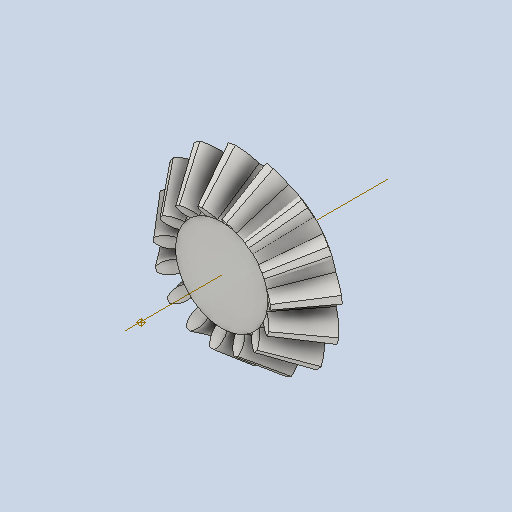
# Autodesk Inventor part: Bevel Gear2
Saved by Autodesk Inventor 2023 (Build 270158000, 158)
## iProperties
Created: 2023-02-02
Part Number: Bevel Gear2
Material: Steel, Mild
Document SubType Name: Modeling
Designer: MOHIKA
Categories: <?xml version="1.0" encoding="UTF-16"?> <MemberInstance><Categories><FamilyTemplate><FamilyTemplateParameter ValueType="xs:double" Id="1" ObjectReferenceKey="da_z" ObjectType="kUserParameterObject"/><FamilyTemplateParameter ValueType="xs:double" Id="2" ObjectReferenceKey="da_b" ObjectType="kUserParameterObject"/><FamilyTemplateParameter ValueType="xs:double" Id="3" ObjectReferenceKey="da_beta" ObjectType="kUserParameterObject"/><FamilyTemplateParameter ValueType="xs:double" Id="4" ObjectReferenceKey="da_dae" ObjectType="kUserParameterObject"/><FamilyTemplateParameter ValueType="xs:double" Id="5" ObjectReferenceKey="da_ve" ObjectType="kUserParameterObject"/><FamilyTemplateParameter ValueType="xs:double" Id="6" ObjectReferenceKey="da_omega" ObjectType="kUserParameterObject"/><FamilyTemplateParameter ValueType="xs:string" Id="7" ObjectReferenceKey="EAIAABAAAAAAHwAAAAAAAIAAAAAAAAAA" ObjectType="83914240" SubObjectId="SurfaceGeometry"/></FamilyTemplate><ParamToTemplateMap><ParamToTemplate CategoryParameter="//CategoryParameter[@InternalName='046C89C9-8512-4d59-83FE-43B91F4F132A']" TemplateParameter="1"/><ParamToTemplate CategoryParameter="//CategoryParameter[@InternalName='2552DF32-E462-4b46-AEBF-C6C7768E72AC']" TemplateParameter="2"/><ParamToTemplate CategoryParameter="//CategoryParameter[@InternalName='C9EE641D-15FC-4fae-A226-E94C4372FDD7']" TemplateParameter="3"/><ParamToTemplate><ParamToTemplate CategoryParameter="//CategoryParameter[@InternalName='00B6519A-459B-49c7-AD84-2E56D39A5744']" ConstantValue="-0.279412"/></ParamToTemplate><ParamToTemplate><ParamToTemplate CategoryParameter="//CategoryParameter[@InternalName='04B31F0E-C7A6-4894-AA32-9629BEFACF47']" ConstantValue="1.000000"/></ParamToTemplate><ParamToTemplate><ParamToTemplate CategoryParameter="//CategoryParameter[@InternalName='43CBEC2E-7847-49e7-A936-2F7889FCB2D9']" ConstantValue="0.200000"/></ParamToTemplate><ParamToTemplate><ParamToTemplate CategoryParameter="//CategoryParameter[@InternalName='B1EFC894-105D-4ebd-86BF-FA20ED196853']" ConstantValue="0.300000"/></ParamToTemplate><ParamToTemplate><ParamToTemplate CategoryParameter="//CategoryParameter[@InternalName='51175063-3D10-4879-93E8-6246FE8B403D']" ConstantValue="2060000000.000000"/></ParamToTemplate><ParamToTemplate><ParamToTemplate CategoryParameter="//CategoryParameter[@InternalName='A3A52E27-4454-46a9-B0BD-C932399B70AF']" ConstantValue="0.300000"/></ParamToTemplate><ParamToTemplate CategoryParameter="//CategoryParameter[@InternalName='2A200944-5A8C-41ca-B96E-8520D2E510F1']" TemplateParameter="4"/><ParamToTemplate><ParamToTemplate CategoryParameter="//CategoryParameter[@InternalName='1A637F62-92C8-44bc-B81F-10802510B579']" ConstantValue="1.557144"/></ParamToTemplate><ParamToTemplate CategoryParameter="//CategoryParameter[@InternalName='B52DD4BE-6863-48fb-BF58-89EF6F9EC65C']" TemplateParameter="5"/><ParamToTemplate><ParamToTemplate CategoryParameter="//CategoryParameter[@InternalName='3956BFF2-84D2-457d-93C2-9B0613DEBA67']" ConstantValue="0.922321"/></ParamToTemplate><ParamToTemplate CategoryParameter="//CategoryParameter[@InternalName='739CFA02-461B-4bf8-8049-181FCAD8B28F']" TemplateParameter="6"/><ParamToTemplate><ParamToTemplate CategoryParameter="//CategoryParameter[@InternalName='A27E999F-E2CE-4481-8A2A-EBF499C4C3C5']" ConstantValue="0.050000"/></ParamToTemplate><ParamToTemplate><ParamToTemplate CategoryParameter="//CategoryParameter[@InternalName='9E1B4470-B2D3-4ff1-B813-535BB4CDF51A']" ConstantValue="3520000.000000"/></ParamToTemplate><ParamToTemplate><ParamToTemplate CategoryParameter="//CategoryParameter[@InternalName='F8452263-BFF6-458c-9FB1-07C4B99E95CD']" ConstantValue="11400000.000000"/></ParamToTemplate><ParamToTemplate><ParamToTemplate CategoryParameter="//CategoryParameter[@InternalName='3E3BB259-FD49-497f-8171-6EBC954A3479']" ConstantValue="2.000000"/></ParamToTemplate><ParamToTemplate CategoryParameter="//CategoryParameter[@InternalName='27C3BAF2-7550-4e4b-AE2C-0DB134B7D9B7']" TemplateParameter="7"/></ParamToTemplateMap><Category DisplayName="Gear" InternalName="DC85795E-93AB-48d5-8EEE-5A27447B64BD" Mnemonic="Gear"><CategoryParameter DisplayName="z" InternalName="046C89C9-8512-4d59-83FE-43B91F4F132A" Mnemonic="z"/><CategoryParameter DisplayName="b" InternalName="2552DF32-E462-4b46-AEBF-C6C7768E72AC" Mnemonic="b"/><CategoryParameter DisplayName="||b|" InternalName="C9EE641D-15FC-4fae-A226-E94C4372FDD7" Mnemonic="beta"/><CategoryParameter DisplayName="x" InternalName="00B6519A-459B-49c7-AD84-2E56D39A5744" Mnemonic="x"/><CategoryParameter DisplayName="a*" InternalName="04B31F0E-C7A6-4894-AA32-9629BEFACF47" Mnemonic="a"/><CategoryParameter DisplayName="c*" InternalName="43CBEC2E-7847-49e7-A936-2F7889FCB2D9" Mnemonic="c"/><CategoryParameter DisplayName="r|.f|*" InternalName="B1EFC894-105D-4ebd-86BF-FA20ED196853" Mnemonic="rf"/><CategoryParameter DisplayName="E" InternalName="51175063-3D10-4879-93E8-6246FE8B403D" Mnemonic="E"/><CategoryParameter DisplayName="||m|" InternalName="A3A52E27-4454-46a9-B0BD-C932399B70AF" Mnemonic="mi"/><Category DisplayName="BevelGear" InternalName="0C98F69A-0C2B-4791-B2FE-7691BB227E77" Mnemonic="BevelGear"><CategoryParameter DisplayName="d|.ae|" InternalName="2A200944-5A8C-41ca-B96E-8520D2E510F1" Mnemonic="dae"/><CategoryParameter DisplayName="d|.ai|" InternalName="1A637F62-92C8-44bc-B81F-10802510B579" Mnemonic="dai"/><CategoryParameter DisplayName="A|.e|" InternalName="B52DD4BE-6863-48fb-BF58-89EF6F9EC65C" Mnemonic="ve"/><CategoryParameter DisplayName="A|.i|" InternalName="3956BFF2-84D2-457d-93C2-9B0613DEBA67" Mnemonic="vi"/><CategoryParameter DisplayName="||S|" InternalName="739CFA02-461B-4bf8-8049-181FCAD8B28F" Mnemonic="omega"/><CategoryParameter DisplayName="x|.t|" InternalName="A27E999F-E2CE-4481-8A2A-EBF499C4C3C5" Mnemonic="xt"/><CategoryParameter DisplayName="||s||.Flim|" InternalName="9E1B4470-B2D3-4ff1-B813-535BB4CDF51A" Mnemonic="sFlim"/><CategoryParameter DisplayName="||s||.Hlim|" InternalName="F8452263-BFF6-458c-9FB1-07C4B99E95CD" Mnemonic="sHlim"/><CategoryParameter DisplayName="type" InternalName="3E3BB259-FD49-497f-8171-6EBC954A3479" Mnemonic="type"/><CategoryParameter DisplayName="PitchDiameter" InternalName="27C3BAF2-7550-4e4b-AE2C-0DB134B7D9B7" Mnemonic="IDS_PITCHDIAM"/></Category></Category></Categories></MemberInstance>
Mass: 60.9118 g
Surface Area: 34.3074 cm^2
Volume: 7.7496 cm^3
Density: 7.86 g/cm^3
Appearance: Steel
CustomPartVersion: 1
Author: MOHIKA
Autodesk Inventor part; units mm, degrees
ref_plane "Mesh Plane2" through (0, 0, 0) normal (0.9781476, 0.2079117, 0) x (0, 0, 1)
sketch "Teeth Body Sketch" plane through (0, 0, 0) normal (1, 0, 0) x (0, 1, 0)
  line L0 (0, 0) -> (9.474706, -16.331471) construction
  line L1 (9.474706, -16.331471) -> (12.114706, -14.351471)
  line L2 (12.114706, -14.351471) -> (0, 0) construction
  line L3 (11.25, -15) -> (0, 0) construction
  line L4 (6.089078, -10.495692) -> (7.785718, -9.223212)
  line L5 (9.474706, -16.331471) -> (6.089078, -10.495692)
  line L6 (12.114706, -14.351471) -> (7.785718, -9.223212)
  line L7 (0, -39.386751) -> (0, 6.564458)
  line L8 (0, -15) -> (12.114706, -15) construction
  dimension "d0" = 22.5
  dimension "d1" = 18.94941
  dimension "d2" = 24.22941
  dimension "d3" = 6.7
  dimension "d4" = 14.35147
  constraints: 16 end point, 4 point on line, 3 perpendicular, 2 collinear, 1 horizontal alignment, 1 vertical alignment
  measures "d0" diameter of L3.start L7
  measures "d1" diameter of L0.end L7
  measures "d2" diameter of L1.end L7
  measures "d3" distance between parallel lines of L1 L4
  measures "d4" vertical distance of L1.end L0.start
revolve "Teeth Body" add sketch "Teeth Body Sketch" angle 360 about axis through (0, 0, 0) along (0, 0, 1)
ref_plane "Tooth Plane" through (0, 11.25, -15) normal (0, -0.6, 0.8) x (1, 0, 0)
sketch "Start Sketch" plane through (0, 11.25, -15) normal (0, -0.6, 0.8) x (1, 0, 0)
  line L0 (0, -23.505131) -> (0, 10.644758)
  arc A0 (-0.947228, -2.615118) -> (-3.205708, 1.749187) centre (-4.944424, -1.917101) ccw
  arc A1 (3.205708, 1.749187) -> (0.947228, -2.615118) centre (4.944424, -1.917101) ccw
  line L1 (-0.947228, -2.615118) -> (0.947228, -2.615118)
  arc A2 (3.205708, 1.749187) -> (-3.205708, 1.749187) centre (0, -14.0625) ccw
  dimension "d7" = 4.05768
  dimension "d8" = 4.94442
  dimension "d9" = 12.1454
  dimension "d57" = 16.13338
  dimension "d58" = 11.44738
  constraints: 6 point on circle, 3 centre point, 3 symmetric about line, 2 end point, 1 coincident, 1 perpendicular, 1 other
  measures "d7" radius of A0
  measures "d8" horizontal distance of point (0, -14.063) A0.centre
  measures "d9" vertical distance of point (0, -14.063) A0.centre
  measures "d57" radius of A2
  measures "d58" distance from line of A2.centre L1
sketch "End Sketch" plane through (0, 7.131, -9.508) normal (0, -0.6, 0.8) x (1, 0, 0)
  line L0 (0, -15.35404) -> (0, 6.953444)
  arc A0 (-0.600416, -1.657636) -> (-2.031992, 1.108752) centre (-3.134106, -1.215187) ccw
  arc A1 (2.031992, 1.108752) -> (0.600416, -1.657636) centre (3.134106, -1.215187) ccw
  line L1 (-0.600416, -1.657636) -> (0.600416, -1.657636)
  arc A2 (2.031992, 1.108752) -> (-2.031992, 1.108752) centre (0, -8.91375) ccw
  dimension "d12" = 2.57203
  dimension "d15" = 3.13411
  dimension "d16" = 7.69856
  dimension "d59" = 10.22641
  dimension "d60" = 7.25611
  constraints: 6 point on circle, 3 centre point, 3 symmetric about line, 2 end point, 1 coincident, 1 other
  measures "d12" radius of A0
  measures "d15" horizontal distance of A0.centre point (0, -8.914)
  measures "d16" vertical distance of A0.centre point (0, -8.914)
  measures "d59" radius of A2
  measures "d60" distance from line of A2.centre L1
loft "Loft" cut profiles "Start Sketch", "End Sketch"
pattern_circular "Circular Pattern" count 15 over 360 about axis through (0, 0, 0) along (0, 0, 1) of "Loft"
ref_plane "End Plane" through (0, 7.131, -9.508) normal (0, -0.6, 0.8) x (1, 0, 0)
sketch3d "3D Sketch Right"
ref_plane "End Plane Right" through (-1.90493, 6.871856, -9.508) normal (0.1602801, -0.5781957, 0.8) x (0.9636595, 0.2671336, 0)
sketch "End Sketch Right" plane through (-1.90493, 6.871856, -9.508) normal (0.1602801, -0.5781957, 0.8) x (0.9636595, 0.2671336, 0)
  arc A0 (-0.600416, -1.657636) -> (-2.031992, 1.108752) centre (-3.134106, -1.215187) ccw
  line L0 (0, -19.153211) -> (0, 10.752604)
  arc A1 (2.031992, 1.108752) -> (0.600416, -1.657636) centre (3.134106, -1.215187) ccw
  line L1 (-0.600416, -1.657636) -> (0.600416, -1.657636)
  arc A2 (2.031992, 1.108752) -> (-2.031992, 1.108752) centre (0, -8.91375) ccw
  dimension "d70" = 3.13411
  dimension "d71" = 7.69856
  dimension "d72" = 2.57203
  dimension "d73" = 7.25611
  dimension "d74" = 10.22641
  constraints: 6 point on circle, 3 centre point, 3 symmetric about line, 2 end point, 1 coincident, 1 perpendicular, 1 other
  measures "d70" horizontal distance of A2.centre A0.centre
  measures "d71" vertical distance of point (0, -8.914) A0.centre
  measures "d72" radius of A0
  measures "d73" distance from line of point (0, -8.914) L1
  measures "d74" radius of A2
feature "Loft Right" [suppressed]
pattern_circular "Circular Pattern Right" [suppressed]
sketch3d "3D Sketch Left"
ref_plane "End Plane Left" through (1.906283, 6.871856, -9.50847) normal (-0.160386, -0.5781669, 0.7999996) x (0.9636106, -0.2673098, 0)
sketch "End Sketch Left" plane through (1.906283, 6.871856, -9.50847) normal (-0.160386, -0.5781669, 0.7999996) x (0.9636106, -0.2673098, 0)
  line L0 (0, -33.290641) -> (0, 16.267917)
  arc A0 (-0.600416, -1.657643) -> (-2.031992, 1.108744) centre (-3.134106, -1.215194) ccw
  arc A1 (2.031992, 1.108744) -> (0.600416, -1.657643) centre (3.134106, -1.215194) ccw
  line L1 (-0.600416, -1.657643) -> (0.600416, -1.657643)
  ellipse E0 centre (0, -5.533932) end of major axis (7.785718, -5.533932) minor radius 6.228571
  arc A2 (2.031992, 1.108744) -> (-2.031992, 1.108744) centre (0, -8.913758) ccw
  dimension "d56" = 6.22857
  dimension "d30" = 2.57203
  dimension "d31" = 3.13411
  dimension "d32" = 7.69856
  dimension "d61" = 10.22641
  dimension "d62" = 7.25611
  constraints: 6 point on circle, 3 centre point, 3 symmetric about line, 2 end point, 1 coincident, 2 other
  measures "d30" radius of A0
  measures "d31" horizontal distance of point (0, -8.914) A0.centre
  measures "d32" vertical distance of A0.centre point (0, -8.914)
  measures "d61" radius of A2
  measures "d62" distance from line of point (0, -8.914) L1
feature "Loft Left" [suppressed]
pattern_circular "Circular Pattern Left" [suppressed]
sketch "Body Sketch" plane through (0, 0, 0) normal (1, 0, 0) x (0, 1, 0)
  line L0 (0, -35.037536) -> (0, -19.530831)
  line L1 (9.474706, -16.331471) -> (6.089078, -10.495692)
  line L2 (6.089078, -10.495692) -> (0, -10.495692)
  line L3 (9.474706, -16.331471) -> (0, -16.331471)
  constraints: 4 end point, 2 perpendicular, 2 point on line
sketch "Body Sketch outline for Fix Body" plane through (0, 0, 0) normal (1, 0, 0) x (0, 1, 0)
  line L0 (0, -16.331471) -> (9.474706, -16.331471)
  line L1 (0, -10.495692) -> (0, -16.331471)
  line L2 (6.089078, -10.495692) -> (0, -10.495692)
  line L3 (9.474706, -16.331471) -> (6.089078, -10.495692)
revolve "Fix Body" add sketch "Body Sketch outline for Fix Body" angle 360 about axis through (0, 0, 0) along (0, 0, 1)
sketch "Sketch6" plane through (0, 0, 0) normal (1, 0, 0) x (0, 1, 0)
  line L0 (11.25, -15) -> (0, 0)
  line L1 (0, -37.799919) -> (0, 6.299986)
surface revolve "Pitch Diameter" sketch "Sketch6" angle 360 about axis through (0, 0, 0) along (0, 0, 1) shown no curves L0
equation "\"d0\" = da_de"
equation "\"d1\" = da_dfe"
equation "\"d2\" = da_dae"
equation "\"d3\" = da_b"
equation "\"d4\" = da_ve"
equation "\"d7\" = fd_rr"
equation "\"d8\" = fd_x"
equation "\"d9\" = fd_y"
equation "\"d57\" = 0.5 * fd_dva + 0.3 * da_he"
equation "\"d58\" = 0.5 * fd_dva - 1.12 * da_he"
equation "\"da_teethtype\" = 0"
equation "\"da_b\" = 6.7"
equation "\"da_de\" = 22.5"
equation "\"da_dae\" = 24.22941"
equation "\"da_dfe\" = 18.94941"
equation "\"da_le\" = 18.75"
equation "\"da_omega\" = 90deg"
equation "\"da_beta\" = 0"
equation "\"da_delta\" = 36.869898deg"
equation "\"da_alpha\" = 20deg"
equation "\"da_he\" = 3.3"
equation "\"da_ve\" = 14.35147"
equation "\"da_zv\" = 18.75"
equation "\"fd_loft\" = da_b + 0.05 * da_he"
equation "\"fd_x\" = fd_x1 + fd_x2"
equation "\"fd_y\" = fd_y1 - fd_y2"
equation "\"fd_dd\" = fd_dva - 0.8 * da_he"
equation "\"da_dvw\" = 27.28676"
equation "\"d11\" = fd_loft"
equation "\"da_dm\" = 18.48"
equation "\"da_x\" = -0.279412"
equation "\"da_m\" = 1.5"
equation "\"d50\" = da_omega"
equation "\"fd_rr\" = 4.057685"
equation "\"fd_dva\" = 30.286765"
equation "\"fd_x1\" = 1.154304"
equation "\"fd_x2\" = 3.790121"
equation "\"fd_y1\" = 13.594465"
equation "\"fd_y2\" = 1.449066"
body "Solid1"
body "Srf1"
